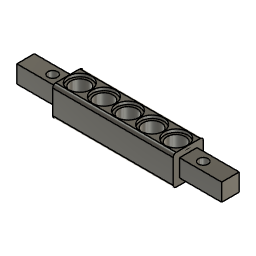
Edge Piece - Cube v1 (Autodesk Fusion 360 design; units mm, degrees)
Autodesk Fusion 360 part; units mm, degrees
sketch "Sketch1" plane through (0, 0, 0) normal (0, 0, 1) x (1, 0, 0)
  line L0 (0, 0) -> (-40, 0)
  line L1 (-40, 0) -> (-40, -10)
  line L2 (-40, -10) -> (0, -10)
  line L3 (0, -10) -> (0, 0)
  dimension "SideLenght" = 40
  dimension "SideWidth" = 10
  constraint horizontal L0
  constraint vertical L1
  constraint horizontal L2
  constraint vertical L3
  constraint coincident L0.start L3.end
  measures "SideLenght" distance of L0.start L0.end
  measures "SideWidth" distance of L0.start L2.end
extrude "Extrude5" add sketch "Sketch1" along normal blind 10
sketch "Sketch5" plane through (0, 0, 0) normal (1, 0, 0) x (0, 1, 0)
  line L0 (-10, 0) -> (0, 0)
  line L1 (0, 0) -> (0, 10)
  line L2 (0, 10) -> (-10, 10)
  line L3 (-10, 10) -> (-10, 0)
  line L4 (-10, 10) -> (-7.9, 10) construction
  line L5 (-7.9, 10) -> (-7.9, 7.9) construction
  line L6 (0, 0) -> (-2.1, 0) construction
  line L7 (-2.1, 0) -> (-2.1, 2.1) construction
  line L8 (-7.9, 7.9) -> (-2.1, 7.9)
  line L9 (-2.1, 7.9) -> (-2.1, 2.1)
  line L10 (-2.1, 2.1) -> (-7.9, 2.1)
  line L11 (-7.9, 2.1) -> (-7.9, 7.9)
  dimension "PegOffset" = 2.1
  dimension "d15" = 2.1
  dimension "d16" = 2.1
  dimension "d17" = 2.1
  constraint coincident L2.end L3.start
  constraint perpendicular L3 L4
  constraint perpendicular L4 L5
  constraint coincident L0.end L1.start
  constraint perpendicular L1 L6
  constraint perpendicular L6 L7
  constraint horizontal L8
  constraint vertical L9
  constraint horizontal L10
  constraint vertical L11
  measures "PegOffset" distance of L2.end L4.end
  measures "d15" distance of L4.end L5.end
  measures "d16" distance of L0.end L6.end
  measures "d17" distance of L6.end L7.end
sketch "Sketch6" plane through (-40, 0, 0) normal (-1, 0, 0) x (0, -1, 0)
  line L0 (0, 0) -> (10, 0)
  line L1 (10, 0) -> (10, 10)
  line L2 (10, 10) -> (0, 10)
  line L3 (0, 10) -> (0, 0)
  line L4 (0, 10) -> (2.1, 10) construction
  line L5 (2.1, 10) -> (2.1, 7.9) construction
  line L6 (10, 0) -> (7.9, 0) construction
  line L7 (7.9, 0) -> (7.9, 2.1) construction
  line L8 (2.1, 7.9) -> (7.9, 7.9)
  line L9 (7.9, 7.9) -> (7.9, 2.1)
  line L10 (7.9, 2.1) -> (2.1, 2.1)
  line L11 (2.1, 2.1) -> (2.1, 7.9)
  dimension "d18" = 2.1
  dimension "d19" = 2.1
  dimension "d20" = 2.1
  dimension "d21" = 2.1
  constraint coincident L2.end L3.start
  constraint coincident L2 L4.end
  constraint perpendicular L4 L5
  constraint coincident L0.end L1.start
  constraint perpendicular L1 L6
  constraint perpendicular L6 L7
  constraint horizontal L8
  constraint vertical L9
  constraint horizontal L10
  constraint vertical L11
  measures "d18" distance of L2.end L4.end
  measures "d19" distance of L4.end L5.end
  measures "d20" distance of L0.end L6.end
  measures "d21" distance of L6.end L7.end
extrude "Extrude6" add sketch "Sketch6" along normal blind 14 contours L8 L9 L10 L11
extrude "Extrude7" add sketch "Sketch5" along normal blind 14 contours L8 L9 L10 L11
sketch "Sketch7" plane through (0, 0, 7.9) normal (0, 0, 1) x (-1, 0, 0)
  line L0 (40, 7.9) -> (40, 2.1)
  line L1 (40, 2.1) -> (54, 2.1)
  line L2 (54, 2.1) -> (54, 7.9)
  line L3 (54, 7.9) -> (40, 7.9)
  line L4 (40, 5) -> (54, 5) construction
  line L5 (40, 5) -> (50, 5) construction
  circle A0 centre (45, 5) radius 1.6
  dimension "d31" = 3.2
  dimension "d33" = 10
  constraint midpoint L0 L4.start
  constraint perpendicular L2 L4
  constraint midpoint L2 L4.end
  constraint midpoint L5 A0.centre
  measures "d31" diameter of A0
  measures "d33" distance of L4.start L5.end
sketch "Sketch8" plane through (0, 0, 7.9) normal (0, 0, 1) x (-1, 0, 0)
  line L0 (0, 2.1) -> (0, 7.9)
  line L1 (0, 7.9) -> (-14, 7.9)
  line L2 (-14, 7.9) -> (-14, 2.1)
  line L3 (-14, 2.1) -> (0, 2.1)
  line L4 (0, 5) -> (-14, 5) construction
  line L5 (-10, 5) -> (0, 5) construction
  circle A0 centre (-5, 5) radius 1.6
  dimension "d32" = 3.2
  dimension "d34" = 10
  constraint midpoint L0 L4.start
  constraint midpoint L2 L4.end
  constraint midpoint L5 A0.centre
  measures "d32" diameter of A0
  measures "d34" distance of L4.start L5.start
extrude "Extrude8" cut sketch "Sketch8" sketch "Sketch7" against normal blind 11 contours A0 of sketch 2 contours A0
fillet "Fillet1" radius 1 1 edges at (-20, 0, 0)
fillet "Fillet1" radius 1 3 edges at (-20, 0, 10) (-20, -10, 10) (-20, -10, 0)
sketch "Sketch9" plane through (0, 0, 10) normal (0, 0, 1) x (-1, 0, 0)
  line L0 (40, 9) -> (0, 9)
  line L1 (0, 9) -> (0, 1)
  line L2 (0, 1) -> (40, 1)
  line L3 (40, 1) -> (40, 9)
  line L4 (20, 1) -> (20, 9) construction
  line L5 (20, 9) -> (40, 9) construction
  line L6 (10, 1) -> (0, 1)
  circle A0 centre (4, 5) radius 4 construction
  line L7 (40, 5) -> (0, 5) construction
  circle A1 centre (12, 5) radius 4 construction
  circle A2 centre (20, 5) radius 4 construction
  circle A3 centre (28, 5) radius 4 construction
  circle A4 centre (4, 5) radius 3.05
  circle A5 centre (12, 5) radius 3.05
  circle A6 centre (36, 5) radius 4 construction
  circle A7 centre (20, 5) radius 3.05
  circle A8 centre (28, 5) radius 3.05
  circle A9 centre (36, 5) radius 3.05
  circle A10 centre (28, 5) radius 3.875
  circle A11 centre (36, 5) radius 3.875
  circle A12 centre (20, 5) radius 3.875
  circle A13 centre (12, 5) radius 3.875
  circle A14 centre (4, 5) radius 3.875
  dimension "d43" = 8
  dimension "d44" = 8
  dimension "d45" = 8
  dimension "d46" = 8
  dimension "d47" = 6.1
  dimension "d48" = 6.1
  dimension "d49" = 8
  dimension "d50" = 6.1
  dimension "d51" = 6.1
  dimension "d52" = 6.1
  dimension "d55" = 7.75
  dimension "d57" = 7.75
  dimension "d58" = 7.75
  dimension "d59" = 7.75
  dimension "d60" = 7.75
  constraint midpoint L2 L4.start
  constraint midpoint L0 L4.end
  constraint coincident L2 L6.start
  constraint coincident L0.start L3.end
  constraint coincident L1.end L2.start
  constraint tangent L1 A0
  constraint midpoint L3 L7.start
  constraint midpoint L1 L7.end
  constraint coincident L7 A1.centre
  constraint tangent A0 A1
  constraint coincident L7 A2.centre
  constraint coincident L7 A3.centre
  constraint tangent A2 A3
  constraint concentric A0 A4
  constraint concentric A1 A5
  constraint tangent A1 A2
  constraint coincident L7 A6.centre
  constraint tangent L3 A6
  constraint concentric A2 A7
  constraint concentric A3 A8
  constraint concentric A6 A9
  constraint coincident A0.centre L7
  constraint concentric A8 A10
  constraint concentric A6 A11
  constraint concentric A7 A12
  constraint concentric A5 A13
  constraint concentric A0 A14
  measures "d43" diameter of A0
  measures "d44" diameter of A1
  measures "d45" diameter of A2
  measures "d46" diameter of A3
  measures "d47" diameter of A4
  measures "d48" diameter of A5
  measures "d49" diameter of A6
  measures "d50" diameter of A7
  measures "d51" diameter of A8
  measures "d52" diameter of A9
  measures "d55" diameter of A10
  measures "d57" diameter of A11
  measures "d58" diameter of A12
  measures "d59" diameter of A13
  measures "d60" diameter of A14
extrude "Extrude9" cut sketch "Sketch9" against normal blind 19 contours A4 | A5 | A7 | A8 | A9
extrude "Extrude10" cut sketch "Sketch9" against normal blind 1 contours A10 | A11 | A12 | A13 | A14
sketch "Sketch10" plane through (0, 0, 0) normal (0, 0, -1) x (1, 0, 0)
  circle A0 centre (-20, 5) radius 3.05
  circle A1 centre (-28, 5) radius 3.05
  circle A2 centre (-4, 5) radius 3.05
  circle A3 centre (-36, 5) radius 3.05
  circle A4 centre (-12, 5) radius 3.05
  line L0 (0, 9) -> (-40, 9)
  line L1 (-40, 9) -> (-40, 1)
  line L2 (-40, 1) -> (0, 1)
  line L3 (0, 1) -> (0, 9)
  circle A5 centre (-4, 5) radius 3.875
  circle A6 centre (-12, 5) radius 3.875
  circle A7 centre (-20, 5) radius 3.875
  circle A8 centre (-28, 5) radius 3.875
  circle A9 centre (-36, 5) radius 3.875
  dimension "d63" = 7.75
  dimension "d64" = 7.75
  dimension "d65" = 7.75
  dimension "d66" = 7.75
  dimension "d67" = 7.75
  constraint concentric A2 A5
  constraint concentric A4 A6
  constraint concentric A0 A7
  constraint concentric A1 A8
  constraint concentric A3 A9
  measures "d63" diameter of A5
  measures "d64" diameter of A6
  measures "d65" diameter of A7
  measures "d66" diameter of A8
  measures "d67" diameter of A9
extrude "Extrude11" cut sketch "Sketch10" against normal blind 1 contours A5 | A6 | A7 | A8 | A9
equation "d12 = SideWidth"
equation "d15 = PegOffset"
equation "d16 = PegOffset"
equation "d17 = PegOffset"
equation "d18 = PegOffset"
equation "d19 = PegOffset"
equation "d20 = PegOffset"
equation "d21 = PegOffset"
equation "PegLenght = 14 mm"
equation "d24 = PegLenght"
equation "PinHole = 6.1 mm"
equation "d47 = PinHole"
equation "d48 = PinHole"
equation "d50 = PinHole"
equation "d51 = PinHole"
equation "d52 = PinHole"
equation "d55 = PinHoleExt"
equation "PinHoleExt = 7.75 mm"
equation "d57 = PinHoleExt"
equation "d58 = PinHoleExt"
equation "d59 = PinHoleExt"
equation "d60 = PinHoleExt"
equation "d63 = PinHoleExt"
equation "d64 = PinHoleExt"
equation "d65 = PinHoleExt"
equation "d66 = PinHoleExt"
equation "d67 = PinHoleExt"
